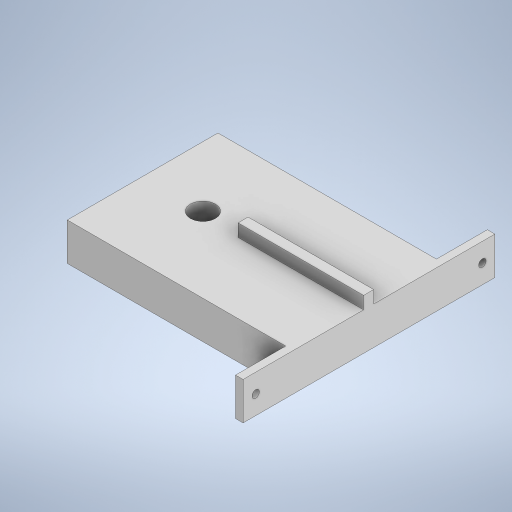
# Autodesk Inventor part: Стенка энкодера штурвала
Saved by Autodesk Inventor 2023 (Build 270158000, 158)
## iProperties
Created: 2022-05-17
Part Number: Стенка энкодера штурвала
Material: Типовые
Document SubType Name: Modeling
Designer: avkap
Density: 1 g/cm^3
Appearance: По умолчанию
Author: avkap
Autodesk Inventor part; units mm, degrees
ref_plane "YZ Plane" through (0, 0, 0) normal (1, 0, 0) x (0, 1, 0)
ref_plane "XZ Plane" through (0, 0, 0) normal (0, 1, 0) x (-1, 0, 0)
ref_plane "XY Plane" through (0, 0, 0) normal (0, 0, 1) x (1, 0, 0)
sketch "Эскиз1" plane through (0, 0, 0) normal (0, 1, 0) x (-1, 0, 0)
  line L0 (0, 0) -> (90, 0)
  line L1 (90, 0) -> (90, -60)
  line L2 (90, -60) -> (0, -60)
  line L3 (0, -60) -> (0, 0)
  line L4 (0, -60) -> (66, -60)
  line L5 (66, -60) -> (66, -30)
  line L6 (66, -30) -> (55, -30)
  line L7 (55, -30) -> (55, -38)
  line L8 (55, -30) -> (55, -22)
  line L9 (55, -22) -> (77, -22)
  line L10 (77, -22) -> (77, -38)
  line L11 (77, -38) -> (55, -38)
  line L12 (0, -60) -> (150, -60)
  line L13 (150, -60) -> (150, 120)
  line L14 (150, 120) -> (0, 120)
  line L15 (0, 120) -> (0, -60)
  point P0 (90, -60)
  dimension "d0" = 90
  dimension "d1" = 60
  dimension "d2" = 66
  dimension "d3" = 30
  dimension "d4" = 11
  dimension "d5" = 8
  dimension "d6" = 8
  dimension "d7" = 22
  dimension "d27" = 150
  dimension "d28" = 180
  constraints: 32 end point, 8 perpendicular, 4 parallel, 2 horizontal, 1 point on line, 1 vertical
  measures "d0" distance of L1.end L2.end
  measures "d1" distance of L0.end L1.end
  measures "d2" distance of L2.end L4.end
  measures "d3" distance of L4.end L5.end
  measures "d4" distance of L5.end L6.end
  measures "d5" distance of L6.end L7.end
  measures "d6" distance of L6.end L8.end
  measures "d7" distance of L8.end L9.end
  measures "d27" distance of L14.end L13.end
  measures "d28" distance of L13.end L12.end
extrude "Выдавливание1" add sketch "Эскиз1" along normal blind 3 contours L0 L1 L2 L3
sketch "Эскиз2" plane through (0, 3, 0) normal (0, 1, 0) x (1, 0, 0)
  line L0 (-90, 60) -> (-90, 0) projected
  line L1 (-90, 0) -> (0, 0)
  line L2 (0, 0) -> (0, 60)
  line L3 (0, 60) -> (-90, 60)
  line L4 (-90, 60) -> (-90, 0)
  circle A0 centre (-66, 30) radius 5
  line L5 (0, 60) -> (-90, 60) projected
  line L6 (0, 60) -> (-150, 60)
  line L7 (-150, 60) -> (-150, -120)
  line L8 (-150, -120) -> (0, -120)
  line L9 (0, -120) -> (0, 60)
  line L10 (-66, 30) -> (0, 30)
  line L11 (0, 0) -> (0, 60) projected
  point P0 (-90, 60)
  dimension "d10" = 10
  dimension "d57" = 66
  constraints: 18 end point, 4 parallel, 2 horizontal, 2 perpendicular, 1 centre point, 1 midpoint
  measures "d10" diameter of A0
  measures "d57" distance of L10.start L10.end
extrude "Выдавливание2" add sketch "Эскиз2" along normal blind 12 contours L3 L2 L1 L0
sketch "Эскиз3" plane through (0, 15, 0) normal (0, 1, 0) x (1, 0, 0)
  line L0 (0, 0) -> (0, 60) projected
  line L1 (0, 30) -> (0, 28)
  line L2 (0, 28) -> (-50, 28)
  line L3 (-50, 28) -> (-50, 32)
  line L4 (-50, 32) -> (0, 32)
  line L5 (0, 32) -> (0, 28)
  point P0 (0, 32)
  dimension "d13" = 2
  dimension "d14" = 50
  dimension "d15" = 4
  constraints: 10 end point, 2 perpendicular, 2 point on line, 1 midpoint
  measures "d13" distance of L1.start L1.end
  measures "d14" distance of L1.end L2.end
  measures "d15" distance of L2.end L3.end
extrude "Выдавливание3" add sketch "Эскиз3" along normal blind 5
sketch "Эскиз6" plane through (0, 15, 0) normal (0, 1, 0) x (1, 0, 0)
  circle A0 centre (-66, 30) radius 5 projected
  line L0 (-66, 30) -> (-66, -120)
  line L1 (-150, -120) -> (0, -120) projected
  line L2 (-66, -120) -> (-66, -100)
  circle A1 centre (-66, -100) radius 10
  circle A2 centre (-66, -100) radius 20
  circle A3 centre (-66, 30) radius 40
  line L3 (-85.7619, -103.0769) -> (-105.5238, 23.8462)
  line L4 (-46.2381, -103.0769) -> (-26.4762, 23.8462)
  line L5 (-66, -100) -> (-66, -40)
  line L6 (-66, -40) -> (-91, -40)
  line L7 (-66, -40) -> (-41, -40)
  circle A4 centre (-91, -40) radius 2.5
  circle A5 centre (-41, -40) radius 2.5
  point P0 (0, 0)
  dimension "d45" = 20
  dimension "d46" = 20
  dimension "d47" = 40
  dimension "d48" = 80
  dimension "d49" = 60
  dimension "d50" = 25
  dimension "d52" = 25
  dimension "d53" = 5
  dimension "d54" = 5
  constraints: 14 end point, 5 centre point, 5 coincident, 4 point on circle, 4 tangent, 3 point on line, 1 perpendicular, 1 vertical
  measures "d45" distance of L0.end L2.end
  measures "d46" diameter of A1
  measures "d47" diameter of A2
  measures "d48" diameter of A3
  measures "d49" distance of L5.start L5.end
  measures "d50" distance of L5.end L6.end
  measures "d52" distance of L5.end L7.end
  measures "d53" diameter of A4
  measures "d54" diameter of A5
sketch "Эскиз7" plane through (0, 0, 0) normal (1, 0, 0) x (0, 0, -1)
  line L0 (80.2787, 0) -> (80.2787, 15)
  line L1 (60, 15) -> (0, 15) projected
  line L2 (80.2787, 15) -> (60.2787, 15)
  line L3 (60.2787, 15) -> (0, 15)
  line L4 (0, 0) -> (0, 15) projected
  line L5 (0, 15) -> (-20, 15)
  line L6 (-20, 15) -> (-20, 0)
  line L7 (-20, 0) -> (0, 0)
  line L8 (-20, 7.5) -> (-15, 7.5)
  line L9 (80.2787, 7.5) -> (75.2787, 7.5)
  circle A0 centre (75.2787, 7.5) radius 1.5
  circle A1 centre (-15, 7.5) radius 1.5
  line L10 (60, 0) -> (0, 0) projected
  line L11 (60, 0) -> (0, 0)
  line L12 (60, 0) -> (60, 15) projected
  line L13 (60, 0) -> (60, 15)
  line L14 (60, 0) -> (80.2787, 0)
  dimension "d59" = 20
  dimension "d60" = 5
  dimension "d61" = 5
  dimension "d62" = 3
  dimension "d63" = 3
  constraints: 22 end point, 4 perpendicular, 3 collinear, 3 horizontal, 2 centre point, 2 coincident, 2 midpoint, 1 point on line
  measures "d59" distance of L1.end L5.end
  measures "d60" distance of L8.start L8.end
  measures "d61" distance of L9.start L9.end
  measures "d62" diameter of A0
  measures "d63" diameter of A1
extrude "Выдавливание7" add sketch "Эскиз7" against normal blind 3
